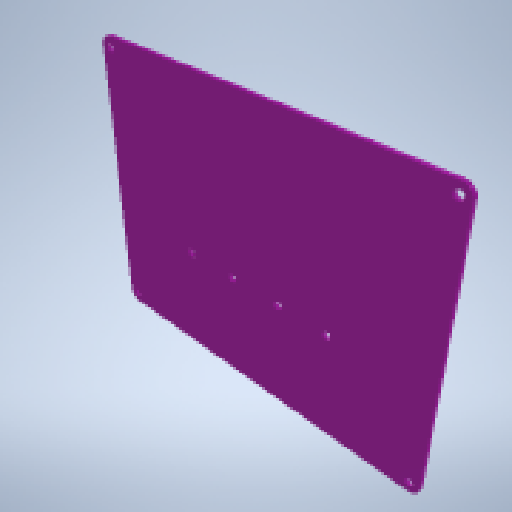
# Autodesk Inventor part: bot_cover_template
Saved by Autodesk Inventor 2024 (Build 280153000, 153)
## iProperties
Created: 2023-11-30
Part Number: bot_cover_template
Material: Generic
Document SubType Name: Modeling
Designer: Ishaan
Density: 1 g/cm^3
Appearance: Smooth - Purple
Author: Ishaan
Autodesk Inventor part; units mm, degrees
ref_plane "YZ Plane" through (0, 0, 0) normal (1, 0, 0) x (0, 1, 0)
ref_plane "XZ Plane" through (0, 0, 0) normal (0, 1, 0) x (-1, 0, 0)
ref_plane "XY Plane" through (0, 0, 0) normal (0, 0, 1) x (1, 0, 0)
sketch "Sketch1" plane through (0, 0, 0) normal (0, 0, 1) x (1, 0, 0)
  line L0 (71.5, -55.5) -> (-71.5, -55.5)
  line L1 (-71.5, -55.5) -> (-71.5, 55.5)
  line L2 (-71.5, 55.5) -> (71.5, 55.5)
  line L3 (71.5, 55.5) -> (71.5, -55.5)
  line L4 (71.5, -55.5) -> (-71.5, 55.5) construction
  line L5 (-71.5, -55.5) -> (71.5, 55.5) construction
  point P0 (0, 0)
  dimension "d0" = 143
  dimension "d1" = 111
  constraints: 12 end point, 2 midpoint, 2 parallel, 1 horizontal, 1 perpendicular
  measures "d0" distance of L1.end L2.end
  measures "d1" distance of L0.end L1.end
extrude "Extrusion1" add sketch "Sketch1" along normal blind 1.6
fillet "Fillet1" radius 4 4 edges at (71.5, 55.5, 0.8) (-71.5, 55.5, 0.8) (-71.5, -55.5, 0.8) (71.5, -55.5, 0.8)
sketch "Sketch2" plane through (0, 0, 1.6) normal (0, 0, 1) x (1, 0, 0)
  arc A0 (67.5, -55.5) -> (71.5, -51.5) centre (67.5, -51.5) ccw projected
  line L0 (71.5, -51.5) -> (71.5, 51.5) projected
  arc A1 (71.5, 51.5) -> (67.5, 55.5) centre (67.5, 51.5) ccw projected
  line L1 (67.5, 55.5) -> (-67.5, 55.5) projected
  arc A2 (-67.5, 55.5) -> (-71.5, 51.5) centre (-67.5, 51.5) ccw projected
  line L2 (-71.5, 51.5) -> (-71.5, -51.5) projected
  arc A3 (-71.5, -51.5) -> (-67.5, -55.5) centre (-67.5, -51.5) ccw projected
  line L3 (-67.5, -55.5) -> (67.5, -55.5) projected
  line L4 (-31.5, -14) -> (31.5, -14) construction
  line L5 (-10.5, -14) -> (10.5, -14) construction
  point P0 (0, 0)
  point P1 (0, -14)
  dimension "d9" = 21
  dimension "d17" = 21
  dimension "d18" = 41.5
  constraints: 8 coincident, 4 end point, 2 midpoint, 2 point on line, 1 horizontal, 1 vertical alignment
  measures "d9" distance of L5.start point (-31.5, -14)
  measures "d17" distance of point (10.5, -14) point (-10.5, -14)
  measures "d18" distance between parallel lines of L3 L4
hole "Hole1" at (-31.5, -14, 1.6) at (31.5, -14, 1.6) at (-10.5, -14, 1.6) at (10.5, -14, 1.6) at (-67.5, 51.5, 1.6) at (67.5, 51.5, 1.6) at (67.5, -51.5, 1.6) at (-67.5, -51.5, 1.6) direction (0, 0, -1) diameter 3.2 end through all
sketch "Sketch3" plane through (0, 0, 1.6) normal (0, 0, 1) x (1, 0, 0)
  line L0 (-67.5, -55.5) -> (67.5, -55.5) projected
  line L1 (-63, -20.5) -> (63, -20.5) construction
  point P0 (0, 0)
  point P1 (-42, -20.5)
  point P2 (-21, -20.5)
  point P3 (0, -20.5)
  point P4 (21, -20.5)
  point P5 (42, -20.5)
  dimension "d21" = 21
  dimension "d26" = 35
  constraints: 2 end point, 2 horizontal, 1 vertical alignment, 6 other
  measures "d21" distance of L1.start point (-42, -20.5)
  measures "d26" distance between parallel lines of L0 L1
sketch "Sketch4" plane through (0, 0, 1.6) normal (0, 0, 1) x (1, 0, 0)
  circle A0 centre (63, -20.5) radius 8 projected
  circle A1 centre (42, -20.5) radius 8 projected
  circle A2 centre (21, -20.5) radius 8 projected
  circle A3 centre (0, -20.5) radius 8 projected
  circle A4 centre (-21, -20.5) radius 8 projected
  circle A5 centre (-42, -20.5) radius 8 projected
  circle A6 centre (-63, -20.5) radius 8 projected
  circle A7 centre (-67.5, -51.5) radius 1.6 projected
  circle A8 centre (67.5, -51.5) radius 1.6 projected
  circle A9 centre (67.5, 51.5) radius 1.6 projected
  circle A10 centre (-67.5, 51.5) radius 1.6 projected
  circle A11 centre (10.5, -14) radius 1.6 projected
  circle A12 centre (-10.5, -14) radius 1.6 projected
  circle A13 centre (31.5, -14) radius 1.6 projected
  circle A14 centre (-31.5, -14) radius 1.6 projected
  arc A15 (67.5, -55.5) -> (71.5, -51.5) centre (67.5, -51.5) ccw projected
  line L0 (71.5, -51.5) -> (71.5, 51.5) projected
  arc A16 (71.5, 51.5) -> (67.5, 55.5) centre (67.5, 51.5) ccw projected
  line L1 (67.5, 55.5) -> (-67.5, 55.5) projected
  arc A17 (-67.5, 55.5) -> (-71.5, 51.5) centre (-67.5, 51.5) ccw projected
  line L2 (-71.5, 51.5) -> (-71.5, -51.5) projected
  arc A18 (-71.5, -51.5) -> (-67.5, -55.5) centre (-67.5, -51.5) ccw projected
  line L3 (-67.5, -55.5) -> (67.5, -55.5) projected
  line L4 (-63, -7.5096) -> (-51.75, -14.0048)
  line L5 (-51.75, -14.0048) -> (-51.75, -26.9952)
  line L6 (-51.75, -26.9952) -> (-63, -33.4904)
  line L7 (-63, -33.4904) -> (-74.25, -26.9952)
  line L8 (-74.25, -26.9952) -> (-74.25, -14.0048)
  line L9 (-74.25, -14.0048) -> (-63, -7.5096)
  line L10 (63, -7.5096) -> (74.25, -14.0048)
  line L11 (74.25, -14.0048) -> (74.25, -26.9952)
  line L12 (74.25, -26.9952) -> (63, -33.4904)
  line L13 (63, -33.4904) -> (51.75, -26.9952)
  line L14 (51.75, -26.9952) -> (51.75, -14.0048)
  line L15 (51.75, -14.0048) -> (63, -7.5096)
  point P0 (0, 0)
  point P1 (71.5, -12.4171)
  point P2 (71.5, -28.5829)
  point P3 (-71.5, -28.5829)
  point P4 (-71.5, -12.4171)
  dimension "d34" = 22.5
  dimension "d35" = 22.5
  constraints: 24 end point, 2 coincident, 2 vertical, 26 other
  measures "d34" distance between parallel lines of L14 L11
  measures "d35" distance between parallel lines of L5 L8
sketch "Sketch5" plane through (0, 0, 1.6) normal (0, 0, 1) x (1, 0, 0)
  line L0 (-42, -6) -> (42, -6) construction
  line L1 (-67.5, -55.5) -> (67.5, -55.5) projected
  circle A0 centre (-42, -20.5) radius 8 projected
  circle A1 centre (-21, -20.5) radius 8 projected
  circle A2 centre (0, -20.5) radius 8 projected
  circle A3 centre (21, -20.5) radius 8 projected
  circle A4 centre (42, -20.5) radius 8 projected
  point P0 (0, 0)
  point P1 (0, -6)
  point P2 (0, -55.5)
  point P3 (-21, -6)
  point P4 (0, -6)
  point P5 (21, -6)
  dimension "d39" = 49.5
  constraints: 7 vertical alignment, 3 midpoint, 3 point on line, 2 end point, 1 coincident, 1 horizontal
  measures "d39" distance between parallel lines of L1 L0
sketch "Sketch6" plane through (0, 0, 1.6) normal (0, 0, 1) x (1, 0, 0)
  line L0 (-67.5, -55.5) -> (67.5, -55.5) construction
  line L1 (-71.5, 51.5) -> (-71.5, -11.2624) construction
  point P0 (0, 0)
  point P1 (-68.5, 13.5)
  point P2 (-63.5, 13.5)
  point P3 (-58.5, 13.5)
  point P4 (-53.5, 13.5)
  dimension "d49" = 5
  dimension "d54" = 69
  dimension "d55" = 3
  constraints: 1 horizontal, 3 other
  measures "d49" distance of point (-68.5, 13.5) point (-63.5, 13.5)
  measures "d54" distance from line of point (-68.5, 13.5) L0
  measures "d55" distance from line of point (-68.5, 13.5) L1
sketch "Sketch7" plane through (0, 0, 1.6) normal (0, 0, 1) x (1, 0, 0)
  circle A0 centre (-68.5, 13.5) radius 1.7 projected
  line L0 (-68.5, 18.1188) -> (-64.5, 15.8094)
  line L1 (-64.5, 15.8094) -> (-64.5, 11.1906)
  line L2 (-64.5, 11.1906) -> (-68.5, 8.8812)
  line L3 (-68.5, 8.8812) -> (-72.5, 11.1906)
  line L4 (-72.5, 11.1906) -> (-72.5, 15.8094)
  line L5 (-72.5, 15.8094) -> (-68.5, 18.1188)
  line L6 (-71.5, 51.5) -> (-71.5, -11.2624) projected
  point P0 (0, 0)
  point P1 (-71.5, 10.6132)
  point P2 (-71.5, 16.3868)
  dimension "d63" = 1
  constraints: 12 end point, 1 coincident, 1 vertical, 13 other
  measures "d63" distance between parallel lines of L6 L4
sketch "Sketch8" plane through (0, 0, 1.6) normal (0, 0, 1) x (1, 0, 0)
  line L0 (68.5, 21.1) -> (34.5, 21.1)
  line L1 (34.5, 21.1) -> (34.5, 40.1)
  line L2 (34.5, 40.1) -> (68.5, 40.1)
  line L3 (68.5, 40.1) -> (68.5, 21.1)
  line L4 (68.5, 21.1) -> (34.5, 40.1) construction
  line L5 (34.5, 21.1) -> (68.5, 40.1) construction
  line L6 (71.5, -11.2624) -> (71.5, 51.5) projected
  line L7 (-67.5, -55.5) -> (67.5, -55.5) projected
  point P0 (0, 0)
  point P1 (51.5, 30.6)
  dimension "d67" = 20
  dimension "d68" = 86.1
  dimension "d69" = 34
  dimension "d70" = 19
  constraints: 12 end point, 2 midpoint, 2 parallel, 1 horizontal, 1 perpendicular
  measures "d67" distance from line of L6 point (51.5, 30.6)
  measures "d68" distance from line of L7 point (51.5, 30.6)
  measures "d69" distance of L1.end L2.end
  measures "d70" distance of L2.end L0.start
sketch "Sketch9" plane through (0, 0, 1.6) normal (0, 0, 1) x (1, 0, 0)
  line L0 (67.25, 14.25) -> (35.75, 14.25)
  line L1 (35.75, 14.25) -> (35.75, 43.95)
  line L2 (35.75, 43.95) -> (67.25, 43.95)
  line L3 (67.25, 43.95) -> (67.25, 14.25)
  line L4 (67.25, 14.25) -> (35.75, 43.95) construction
  line L5 (35.75, 14.25) -> (67.25, 43.95) construction
  line L6 (-67.5, -55.5) -> (67.5, -55.5) projected
  point P0 (0, 0)
  point P1 (51.5, 29.1)
  point P2 (51.5, 30.6)
  dimension "d74" = 31.5
  dimension "d75" = 29.7
  dimension "d76" = 69.75
  constraints: 12 end point, 4 coincident, 2 midpoint, 2 parallel, 1 horizontal, 1 perpendicular, 1 vertical alignment
  measures "d74" distance of L1.end L2.end
  measures "d75" distance of L2.end L0.start
  measures "d76" distance between parallel lines of L6 L0
sketch "Sketch10" plane through (0, 0, 1.6) normal (0, 0, 1) x (1, 0, 0)
  circle A0 centre (35.75, 14.25) radius 3 projected
  circle A1 centre (67.25, 14.25) radius 3 projected
  circle A2 centre (67.25, 43.95) radius 3 projected
  circle A3 centre (35.75, 43.95) radius 3 projected
  line L0 (34.5, 22.1) -> (34.5, 39.1) projected
  arc A4 (35.5, 40.1) -> (34.5, 39.1) centre (35.5, 39.1) ccw projected
  line L1 (35.5, 40.1) -> (67.5, 40.1) projected
  arc A5 (68.5, 39.1) -> (67.5, 40.1) centre (67.5, 39.1) ccw projected
  line L2 (68.5, 39.1) -> (68.5, 22.1) projected
  arc A6 (67.5, 21.1) -> (68.5, 22.1) centre (67.5, 22.1) ccw projected
  line L3 (67.5, 21.1) -> (35.5, 21.1) projected
  arc A7 (34.5, 22.1) -> (35.5, 21.1) centre (35.5, 22.1) ccw projected
  circle A8 centre (-53.5, 13.5) radius 1.7 projected
  circle A9 centre (-58.5, 13.5) radius 1.7 projected
  circle A10 centre (-63.5, 13.5) radius 1.7 projected
  circle A11 centre (-68.5, 13.5) radius 1.7 projected
  circle A12 centre (42, -6) radius 2.75 projected
  circle A13 centre (21, -6) radius 2.75 projected
  circle A14 centre (0, -6) radius 2.75 projected
  circle A15 centre (-21, -6) radius 2.75 projected
  circle A16 centre (-42, -6) radius 2.75 projected
  circle A17 centre (63, -20.5) radius 8 projected
  circle A18 centre (42, -20.5) radius 8 projected
  circle A19 centre (21, -20.5) radius 8 projected
  circle A20 centre (0, -20.5) radius 8 projected
  circle A21 centre (-21, -20.5) radius 8 projected
  circle A22 centre (-42, -20.5) radius 8 projected
  circle A23 centre (-63, -20.5) radius 8 projected
  circle A24 centre (-67.5, -51.5) radius 1.6 projected
  circle A25 centre (67.5, -51.5) radius 1.6 projected
  circle A26 centre (67.5, 51.5) radius 1.6 projected
  circle A27 centre (-67.5, 51.5) radius 1.6 projected
  circle A28 centre (10.5, -14) radius 1.6 projected
  circle A29 centre (-10.5, -14) radius 1.6 projected
  circle A30 centre (31.5, -14) radius 1.6 projected
  circle A31 centre (-31.5, -14) radius 1.6 projected
  arc A32 (-72.5, 11.6236) -> (-72.125, 10.9741) centre (-71.75, 11.6236) ccw projected
  line L4 (-72.125, 10.9741) -> (-71.875, 10.8298) projected
  arc A33 (-71.5, 10.1802) -> (-71.875, 10.8298) centre (-72.25, 10.1802) ccw projected
  line L5 (-71.5, 10.1802) -> (-71.5, -11.2624) projected
  arc A34 (-72.5, -12.9944) -> (-71.5, -11.2624) centre (-73.5, -11.2624) ccw projected
  line L6 (-72.5, -12.9944) -> (-73.25, -13.4275) projected
  arc A35 (-73.25, -13.4275) -> (-74.25, -15.1595) centre (-72.25, -15.1595) ccw projected
  line L7 (-74.25, -15.1595) -> (-74.25, -25.8405) projected
  arc A36 (-74.25, -25.8405) -> (-73.25, -27.5725) centre (-72.25, -25.8405) ccw projected
  line L8 (-73.25, -27.5725) -> (-72.5, -28.0056) projected
  arc A37 (-71.5, -29.7376) -> (-72.5, -28.0056) centre (-73.5, -29.7376) ccw projected
  line L9 (-71.5, -29.7376) -> (-71.5, -51.5) projected
  arc A38 (-71.5, -51.5) -> (-67.5, -55.5) centre (-67.5, -51.5) ccw projected
  line L10 (-67.5, -55.5) -> (67.5, -55.5) projected
  arc A39 (67.5, -55.5) -> (71.5, -51.5) centre (67.5, -51.5) ccw projected
  line L11 (71.5, -51.5) -> (71.5, -29.7376) projected
  arc A40 (72.5, -28.0056) -> (71.5, -29.7376) centre (73.5, -29.7376) ccw projected
  line L12 (72.5, -28.0056) -> (73.25, -27.5725) projected
  arc A41 (73.25, -27.5725) -> (74.25, -25.8405) centre (72.25, -25.8405) ccw projected
  line L13 (74.25, -25.8405) -> (74.25, -15.1595) projected
  arc A42 (74.25, -15.1595) -> (73.25, -13.4275) centre (72.25, -15.1595) ccw projected
  line L14 (73.25, -13.4275) -> (72.5, -12.9944) projected
  arc A43 (71.5, -11.2624) -> (72.5, -12.9944) centre (73.5, -11.2624) ccw projected
  line L15 (71.5, -11.2624) -> (71.5, 51.5) projected
  arc A44 (71.5, 51.5) -> (67.5, 55.5) centre (67.5, 51.5) ccw projected
  line L16 (67.5, 55.5) -> (-67.5, 55.5) projected
  arc A45 (-67.5, 55.5) -> (-71.5, 51.5) centre (-67.5, 51.5) ccw projected
  line L17 (-71.5, 51.5) -> (-71.5, 16.8198) projected
  arc A46 (-71.875, 16.1702) -> (-71.5, 16.8198) centre (-72.25, 16.8198) ccw projected
  line L18 (-71.875, 16.1702) -> (-72.125, 16.0259) projected
  arc A47 (-72.125, 16.0259) -> (-72.5, 15.3764) centre (-71.75, 15.3764) ccw projected
  line L19 (-72.5, 15.3764) -> (-72.5, 11.6236) projected
  line L20 (67.25, 21.4669) -> (73.5, 17.8584)
  line L21 (73.5, 17.8584) -> (73.5, 10.6416)
  line L22 (73.5, 10.6416) -> (67.25, 7.0331)
  line L23 (67.25, 7.0331) -> (61, 10.6416)
  line L24 (61, 10.6416) -> (61, 17.8584)
  line L25 (61, 17.8584) -> (67.25, 21.4669)
  line L26 (67.25, 51.1669) -> (73.5, 47.5584)
  line L27 (73.5, 47.5584) -> (73.5, 40.3416)
  line L28 (73.5, 40.3416) -> (67.25, 36.7331)
  line L29 (67.25, 36.7331) -> (61, 40.3416)
  line L30 (61, 40.3416) -> (61, 47.5584)
  line L31 (61, 47.5584) -> (67.25, 51.1669)
  line L32 (73.5, 40.3416) -> (73.5, 17.8584)
  point P0 (0, 0)
  point P1 (71.5, 48.7131)
  point P2 (71.5, 9.4869)
  dimension "d84" = 2
  constraints: 26 end point, 2 coincident, 2 collinear, 2 vertical, 26 other
  measures "d84" distance between parallel lines of L15 L32
equation "\"d9\" = d8"
equation "\"d35\" = d34"
equation "\"d8\" = 21"
body "Solid1"
